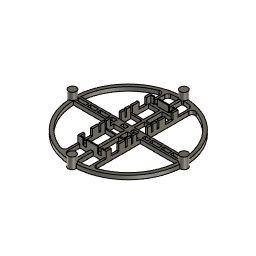
Upper_Bulkhead (Autodesk Fusion 360 design; units mm, degrees)
Autodesk Fusion 360 part; units mm, degrees
sketch "Sketch1" plane through (0, 0, 0) normal (0, 0, 1) x (1, 0, 0)
  circle A0 centre (-0.0658, -87) radius 6
  circle A1 centre (-0.0091, -87) radius 3.15
  circle A2 centre (0.0017, 0.5072) radius 87
  circle A3 centre (-86.9982, 0.5525) radius 3.15
  circle A4 centre (-86.9982, 0.5525) radius 6
  circle A5 centre (87, -0.0091) radius 6
  circle A6 centre (87, -0.0091) radius 3.15
  circle A7 centre (0.0091, 87) radius 3.15
  circle A8 centre (-0.0658, 87) radius 6
  circle A9 centre (0.0017, 0.5072) radius 72.5
  line L0 (-3.9982, 75.5616) -> (4.0018, 75.5616)
  line L1 (4.0018, 75.5616) -> (4.0018, -76.3795)
  line L2 (4.0018, -76.3795) -> (-3.9982, -76.3795)
  line L3 (-3.9982, -76.3795) -> (-3.9982, 75.5616)
  line L4 (-19.9982, 74.1543) -> (-11.9982, 74.1543)
  line L5 (-11.9982, 74.1543) -> (-11.9982, -70.9928)
  line L6 (-11.9982, -70.9928) -> (-19.9982, -70.9928)
  line L7 (-19.9982, -70.9928) -> (-19.9982, 74.1543)
  line L8 (12.0018, -70.9928) -> (20.0018, -70.9928)
  line L9 (20.0018, -70.9928) -> (20.0018, 75.5068)
  line L10 (20.0018, 75.5068) -> (12.0018, 75.5068)
  line L11 (12.0018, 75.5068) -> (12.0018, -70.9928)
  line L12 (0, 2.5) -> (0, 20)
  line L13 (-76.1815, -3) -> (75.8451, -3)
  line L14 (75.8451, -3) -> (75.8451, 0)
  line L15 (75.8451, 0) -> (-76.1815, 0)
  line L16 (-76.1815, 0) -> (-76.1815, -3)
  circle A10 centre (0.0017, 0.5072) radius 82
  line L17 (75.8451, -3) -> (81.9267, -3)
  line L18 (75.8451, 0) -> (82.0002, 0)
  line L19 (20.0018, -70.9928) -> (20.0018, -79.0164)
  line L20 (12.0018, -70.9928) -> (12.0018, -80.61)
  line L21 (-11.9982, -70.9928) -> (-11.9982, -80.61)
  line L22 (-3.9982, -76.3795) -> (-3.9982, -81.3952)
  line L23 (4.0018, -76.3795) -> (4.0018, -81.3952)
  line L24 (-19.9982, -70.9928) -> (-19.9982, -79.0164)
  line L25 (-19.9982, 74.1543) -> (-19.9982, 80.0307)
  line L26 (-11.9982, 74.1543) -> (-11.9982, 81.6244)
  line L27 (-3.9982, 75.5616) -> (-3.9982, 82.4095)
  line L28 (4.0018, 75.5616) -> (4.0018, 82.4095)
  line L29 (12.0018, 75.5068) -> (12.0018, 81.6244)
  line L30 (-76.1815, -3) -> (-81.9232, -3)
  line L31 (-81.9967, 0) -> (-76.1815, 0)
  line L32 (81.8786, 5) -> (-81.8751, 5)
  line L33 (81.6587, 8) -> (-81.6552, 8)
  line L34 (20.0018, 75.5068) -> (20.0018, 80.0307)
  line L35 (66.0018, 0) -> (66.0018, 5)
  line L36 (63.0018, 5) -> (63.0018, 0)
  line L37 (51.0018, 0) -> (51.0018, 5)
  line L38 (48.0018, 0) -> (48.0018, 5)
  line L39 (33.0018, 5) -> (33.0018, 0)
  line L40 (30.0018, 0) -> (30.0018, 5)
  line L41 (-30.0018, 0) -> (-30.0018, 5)
  line L42 (-33.0018, 5) -> (-33.0018, 0)
  line L43 (-48.0018, 0) -> (-48.0018, 5)
  line L44 (-51.0018, 0) -> (-51.0018, 5)
  line L45 (-63.0018, 5) -> (-63.0018, 0)
  line L46 (-66.0018, 0) -> (-66.0018, 5)
  dimension "d15" = 6.3
  dimension "d16" = 12
  dimension "d28" = 6.3
  dimension "d29" = 12
  dimension "d31" = 12
  dimension "d33" = 12
  dimension "d7" = 174
  dimension "d8" = 145
  dimension "d9" = 8
  dimension "d11" = 8
  dimension "d12" = 8
  dimension "d13" = 8
  dimension "d14" = 67
  dimension "d17" = 87
  dimension "d19" = 8
  dimension "d30" = 6.3
  dimension "d32" = 6.3
  dimension "d41" = 3
  dimension "d42" = 3
  dimension "d51" = 164
  dimension "d52" = 5
  dimension "d53" = 3
  dimension "d54" = 3
  dimension "d55" = 3
  dimension "d56" = 3
  dimension "d57" = 15
  dimension "d58" = 15
  dimension "d60" = 10
  constraint concentric A5 A6
  constraint concentric A3 A4
  constraint coincident A3.centre A2
  constraint concentric A2 A9
  constraint horizontal L0
  constraint vertical L1
  constraint horizontal L2
  constraint vertical L3
  constraint horizontal L4
  constraint vertical L5
  constraint horizontal L6
  constraint vertical L7
  constraint coincident A9 L5.end
  constraint horizontal L8
  constraint vertical L9
  constraint horizontal L10
  constraint vertical L11
  constraint coincident A9 L8.start
  constraint horizontal L13
  constraint vertical L14
  constraint horizontal L15
  constraint vertical L16
  constraint concentric A9 A10
  constraint coincident A10 L17.end
  constraint perpendicular L14 L17
  constraint coincident A10 L18.end
  constraint perpendicular L14 L18
  constraint coincident A10 L19.end
  constraint perpendicular L8 L19
  constraint coincident A10 L20.end
  constraint perpendicular L8 L20
  constraint coincident A10 L21.end
  constraint perpendicular L6 L21
  constraint coincident A10 L22.end
  constraint perpendicular L2 L22
  constraint coincident A10 L23.end
  constraint perpendicular L2 L23
  constraint coincident A10 L24.end
  constraint perpendicular L6 L24
  constraint coincident A10 L25.end
  constraint perpendicular L4 L25
  constraint coincident A10 L26.end
  constraint perpendicular L4 L26
  constraint coincident A10 L27.end
  constraint perpendicular L0 L27
  constraint coincident A10 L28.end
  constraint perpendicular L0 L28
  constraint coincident A10 L29.end
  constraint perpendicular L10 L29
  constraint coincident A10 L30.end
  constraint perpendicular L16 L30
  constraint coincident A10 L31.start
  constraint perpendicular L16 L31
  constraint coincident A10 L32.start
  constraint coincident A10 L32.end
  constraint coincident A10 L33.start
  constraint coincident A10 L33.end
  constraint coincident A10 L34.end
  constraint perpendicular L10 L34
  constraint coincident L15 L35.start
  constraint coincident L32 L35.end
  constraint perpendicular L32 L35
  constraint coincident L32 L36.start
  constraint coincident L15 L36.end
  constraint perpendicular L15 L36
  constraint coincident L15 L37.start
  constraint coincident L32 L37.end
  constraint perpendicular L32 L37
  constraint coincident L15 L38.start
  constraint coincident L32 L38.end
  constraint perpendicular L32 L38
  constraint coincident L32 L39.start
  constraint coincident L15 L39.end
  constraint perpendicular L32 L39
  constraint coincident L15 L40.start
  constraint coincident L32 L40.end
  constraint perpendicular L32 L40
  constraint symmetric L12 L35.start L46.start
  constraint symmetric L12 L35.end L46.end
  constraint symmetric L12 L36.start L45.start
  constraint symmetric L12 L36.end L45.end
  constraint symmetric L12 L37.start L44.start
  constraint symmetric L12 L37.end L44.end
  constraint symmetric L12 L38.start L43.start
  constraint symmetric L12 L38.end L43.end
  constraint symmetric L12 L39.start L42.start
  constraint symmetric L12 L39.end L42.end
  constraint symmetric L12 L40.start L41.start
  constraint symmetric L12 L40.end L41.end
  measures "d15" diameter of A6
  measures "d16" diameter of A5
  measures "d28" diameter of A3
  measures "d29" diameter of A4
  measures "d31" diameter of A0
  measures "d33" diameter of A8
  measures "d7" diameter of A2
  measures "d8" diameter of A9
  measures "d9" distance of L1 L3
  measures "d11" distance of L5 L7
  measures "d12" distance of L9 L11
  measures "d13" distance of L3 L5
  measures "d14" distance of A3.centre L7
  measures "d17" distance of origin A3.centre
  measures "d19" distance of L1 L11
  measures "d30" diameter of A1
  measures "d32" diameter of A7
  measures "d41" distance of L13 L15
  measures "d42" distance of origin L13
  measures "d51" diameter of A10
  measures "d52" distance of L15 L32
  measures "d53" distance of L32 L33
  measures "d54" distance of L35 L36
  measures "d55" distance of L37 L38
  measures "d56" distance of L39 L40
  measures "d57" distance of L38 L39
  measures "d58" distance of L35 L37
  measures "d60" distance of L9 L40
extrude "Extrude1" add sketch "Sketch1" along normal blind 6 contours A0 A1 A2 | A0 A1 A2 A10 | A0 A2 A5 A10 | A0 A2 A4 A10 | A0 A10 | A2 A5 A6 A10 | A2 A5 A6 | A2 A3 A4 | A2 A3 A4 A10 | A5 A10 L17 | A2 A4 A8 A10 | A4 A10 L31 | A4 L16 A10 L30 L31 | A5 L14 L17 L18 | A5 A10 L17 L18 | A2 A5 A8 A10 | A2 A7 A8 | A2 A7 A8 A10 | A4 A10 L31 | A5 A10 L18 | A9 L13 L14 L15 | A8 A10 | A9 A10 L32 L33 | A9 L13 L15 L16 | L1 L11 L13 L15 | L9 L11 L13 L15 | L1 L3 L13 L15 | A9 L9 L13 L15 | A9 A10 L32 L33 | L5 L7 L13 L15 | L3 L5 L13 L15 | A9 L7 L32 L33 | A9 L7 L13 L15 | L9 L11 L15 L32 | L1 L3 L15 L32 | A9 L9 L32 L33 | L5 L7 L15 L32 | L15 L32 L45 L46 | L1 L11 L32 L33 | L9 L11 L32 L33 | L1 L12 L32 L33 | L15 L32 L35 L36 | L5 L7 L32 L33 | L3 L5 L32 L33 | L3 L12 L32 L33 | L15 L32 L39 L40 | L15 L32 L41 L42 | L15 L32 L43 L44 | L15 L32 L37 L38
extrude "Extrude2" add sketch "Sketch1" along normal blind 2 contours A0 A1 A2 | A0 A1 A2 A10 | A0 A10 | A2 A5 A6 A10 | A2 A5 A6 | A2 A3 A4 | A2 A3 A4 A10 | A5 A10 L17 | A4 A10 L31 | A5 A10 L17 L18 | A2 A7 A8 | A2 A7 A8 A10 | A4 A10 L31 | A5 A10 L18 | A8 A10
extrude "Extrude3" add sketch "Sketch1" along normal blind 10 contours A0 A1 A2 | A0 A1 A2 A10 | A0 A10 | A2 A5 A6 A10 | A2 A5 A6 | A2 A3 A4 | A2 A3 A4 A10 | A5 A10 L17 | A4 A10 L31 | A5 A10 L17 L18 | A2 A7 A8 | A2 A7 A8 A10 | A4 A10 L31 | A5 A10 L18 | A8 A10
extrude "Extrude4" add sketch "Sketch1" along normal blind 7 from surface at 10 contours A0 A1 A2 | A0 A1 A2 A10 | A0 A10 | A1 A2 | A1 A2 | A2 A5 A6 A10 | A2 A5 A6 | A2 A3 A4 | A2 A3 A4 A10 | A2 A6 | A2 A6 | A5 A10 L17 | A2 A3 | A2 A3 | A4 A10 L31 | A5 A10 L17 L18 | A2 A7 A8 | A2 A7 A8 A10 | A4 A10 L31 | A5 A10 L18 | A2 A7 | A2 A7 | A8 A10
sketch "Sketch2" plane through (0, 0, 6) normal (0, 0, 1) x (-1, 0, 0)
  arc A0 (-81, 0) -> (-81.7986, 3) centre (-87, 0.0091) ccw
  arc A1 (-3.8087, -82.4187) -> (-5.9264, -87.3052) centre (0.0658, -87) ccw
  arc A2 (6.0585, -87.2958) -> (86.7882, -6.5489) centre (-0.0017, -0.5072) ccw
  arc A3 (81.9333, -3.7692) -> (86.7882, -6.5489) centre (86.9982, -0.5525) ccw
  line L0 (-19, 54.5) -> (19, 54.5)
  line L1 (19, 54.5) -> (19, -54.5)
  line L2 (19, -54.5) -> (-19, -54.5)
  line L3 (-19, -54.5) -> (-19, 54.5)
  line L4 (-20.0018, -55.9949) -> (19.9982, -55.9949)
  line L5 (19.9982, -50.9756) -> (19.9982, -55.9949)
  line L6 (19.9982, -50.9756) -> (-20.0018, -50.9756)
  line L7 (-20.0018, -50.9756) -> (-20.0018, -55.9949)
  line L8 (-1.75, 0) -> (-22.5, 0)
  line L9 (19.9982, 50.9756) -> (-20.0018, 50.9756)
  line L10 (-20.0018, 50.9756) -> (-20.0018, 55.9949)
  line L11 (19.9982, 50.9756) -> (19.9982, 55.9949)
  line L12 (-20.0018, 55.9949) -> (19.9982, 55.9949)
  line L13 (-20.0018, -50.9756) -> (-20.0018, 55.9949)
  line L14 (19.9982, 55.9949) -> (19.9982, -50.9756)
  line L15 (19.9982, -55.9949) -> (22.0168, -55.9949)
  line L16 (22.0168, -55.9949) -> (22.0168, 55.9949)
  line L17 (22.0168, 55.9949) -> (19.9982, 55.9949)
  line L18 (0, -1.75) -> (0, -22.5)
  line L19 (-22.0168, -55.9949) -> (-22.0168, 55.9949)
  line L20 (-19.9982, -55.9949) -> (-22.0168, -55.9949)
  line L21 (-22.0168, 55.9949) -> (-19.9982, 55.9949)
  line L22 (-19, -48.1115) -> (-22.0168, -48.1115)
  line L23 (-19, -36.3655) -> (-22.0168, -36.3655)
  line L24 (-19, -32.5412) -> (-22.0168, -32.5412)
  line L25 (-19, -26.0763) -> (-22.0168, -26.0763)
  line L26 (-19, -23.3447) -> (-22.0168, -23.3447)
  line L27 (-19, -16.6067) -> (-22.0168, -16.6067)
  line L28 (-19, -14.6035) -> (-22.0168, -14.6035)
  line L29 (-19, -8.3319) -> (-22.0168, -8.3319)
  line L30 (-19, -6.0084) -> (-22.0168, -6.0084)
  line L31 (19, -32.5412) -> (22.0168, -32.5412)
  line L32 (19, -26.0763) -> (22.0168, -26.0763)
  line L33 (19, -23.3447) -> (22.0168, -23.3447)
  line L34 (19, -36.3655) -> (22.0168, -36.3655)
  line L35 (19, -48.1115) -> (22.0168, -48.1115)
  line L36 (19, -16.6067) -> (22.0168, -16.6067)
  line L37 (19, -14.6035) -> (22.0168, -14.6035)
  line L38 (19, -8.3319) -> (22.0168, -8.3319)
  line L39 (19, -6.0084) -> (22.0168, -6.0084)
  line L40 (-19, 48.1115) -> (-22.0168, 48.1115)
  line L41 (-19, 36.3655) -> (-22.0168, 36.3655)
  line L42 (-19, 32.5412) -> (-22.0168, 32.5412)
  line L43 (-19, 26.0763) -> (-22.0168, 26.0763)
  line L44 (-19, 23.3447) -> (-22.0168, 23.3447)
  line L45 (-19, 16.6067) -> (-22.0168, 16.6067)
  line L46 (-19, 14.6035) -> (-22.0168, 14.6035)
  line L47 (-19, 8.3319) -> (-22.0168, 8.3319)
  line L48 (-19, 6.0084) -> (-22.0168, 6.0084)
  line L49 (19, 6.0084) -> (22.0168, 6.0084)
  line L50 (19, 8.3319) -> (22.0168, 8.3319)
  line L51 (19, 14.6035) -> (22.0168, 14.6035)
  line L52 (19, 16.6067) -> (22.0168, 16.6067)
  line L53 (19, 23.3447) -> (22.0168, 23.3447)
  line L54 (19, 26.0763) -> (22.0168, 26.0763)
  line L55 (19, 32.5412) -> (22.0168, 32.5412)
  line L56 (19, 36.3655) -> (22.0168, 36.3655)
  line L57 (19, 48.1115) -> (22.0168, 48.1115)
  arc A4 (-81.9562, -3.2405) -> (-81.8786, -5) centre (-0.0017, -0.5072) ccw
  line L58 (-81.6587, -8) -> (81.6552, -8)
  line L59 (3.9982, -5) -> (3.9982, 0)
  line L60 (-81, 0) -> (-66.0018, 0)
  line L61 (11.9982, 0) -> (11.9982, -5)
  line L62 (11.9982, -5) -> (3.9982, -5)
  line L63 (-51.0018, -5) -> (-63.0018, -5)
  line L64 (19.9982, -5) -> (19.9982, 0)
  line L65 (81.9232, 3) -> (-81.7986, 3)
  line L66 (-30.0018, 0) -> (-20.0018, 0)
  line L67 (-20.0018, 0) -> (-20.0018, -5)
  line L68 (-12.0018, -5) -> (-12.0018, 0)
  line L69 (-12.0018, 0) -> (-4.0018, 0)
  line L70 (-4.0018, 0) -> (-4.0018, -5)
  line L71 (-4.0018, -5) -> (-12.0018, -5)
  line L72 (19.9982, 0) -> (30.0018, 0)
  line L73 (81.8751, -5) -> (66.0018, -5)
  arc A5 (2.3665, 81.4586) -> (6.0229, 86.284) centre (0.0658, 87) ccw
  arc A6 (-86.8289, -5.9884) -> (-5.9264, -87.3052) centre (-0.0017, -0.5072) ccw
  arc A7 (86.7945, 5.444) -> (6.0229, 86.284) centre (-0.0017, -0.5072) ccw
  line L74 (-63.0018, -5) -> (-63.0018, 0)
  line L75 (-51.0018, 0) -> (-51.0018, -5)
  line L76 (-48.0018, -5) -> (-48.0018, 0)
  line L77 (-48.0018, 0) -> (-33.0018, 0)
  line L78 (-33.0018, 0) -> (-33.0018, -5)
  line L79 (-66.0018, 0) -> (-66.0018, -5)
  line L80 (-30.0018, -5) -> (-30.0018, 0)
  arc A8 (81.9232, 3) -> (2.3665, 81.4586) centre (-0.0017, -0.5072) ccw
  line L81 (51.0018, -5) -> (51.0018, 0)
  line L82 (51.0018, 0) -> (63.0018, 0)
  line L83 (63.0018, 0) -> (63.0018, -5)
  line L84 (63.0018, -5) -> (51.0018, -5)
  line L85 (66.0018, 0) -> (81.0237, 0)
  line L86 (66.0018, -5) -> (66.0018, 0)
  line L87 (48.0018, -5) -> (33.0018, -5)
  line L88 (33.0018, -5) -> (33.0018, 0)
  line L89 (33.0018, 0) -> (48.0018, 0)
  line L90 (48.0018, 0) -> (48.0018, -5)
  line L91 (30.0018, 0) -> (30.0018, -5)
  line L92 (30.0018, -5) -> (19.9982, -5)
  arc A9 (3.9332, -82.4127) -> (81.6552, -8) centre (-0.0017, -0.5072) ccw
  line L93 (-63.0018, 0) -> (-51.0018, 0)
  line L94 (-33.0018, -5) -> (-48.0018, -5)
  line L95 (-66.0018, -5) -> (-81.8786, -5)
  line L96 (-20.0018, -5) -> (-30.0018, -5)
  arc A10 (-86.8289, -5.9884) -> (-81.9562, -3.2405) centre (-87, 0.0091) ccw
  arc A11 (-81.6587, -8) -> (-3.8087, -82.4187) centre (-0.0017, -0.5072) ccw
  arc A12 (6.0585, -87.2958) -> (3.9332, -82.4127) centre (0.0658, -87) ccw
  arc A13 (81.8751, -5) -> (81.9333, -3.7692) centre (-0.0017, -0.5072) ccw
  arc A14 (86.7945, 5.444) -> (81.0237, 0) centre (86.9982, -0.5525) ccw
  line L97 (3.9982, 0) -> (11.9982, 0)
  line L98 (-19, -54.5) -> (-19, -80.276)
  line L99 (-22.0168, -55.9949) -> (-22.0168, -79.4966)
  line L100 (22.0168, -55.9949) -> (22.0168, -79.4957)
  line L101 (19, -54.5) -> (19, -80.2752)
  line L102 (22.0168, 55.9949) -> (22.0168, 78.4813)
  line L103 (19, 54.5) -> (19, 79.2608)
  line L104 (-19, 54.5) -> (-19, 79.2608)
  line L105 (-22.0168, 55.9949) -> (-22.0168, 79.2608)
  line L106 (-22.0168, 79.2608) -> (-19, 79.2608)
  line L107 (-2, 6.1969) -> (-2, -11.5663)
  line L108 (2, 6.1969) -> (2, -11.6219)
  line L109 (2, -11.6219) -> (-2, -11.5663)
  line L110 (-2, 6.1969) -> (2, 6.1969)
  line L111 (-2, -11.5663) -> (1.9507, -11.5663)
  line L112 (1.9507, -11.5663) -> (1.9507, -82.4127)
  line L113 (1.9507, -82.4127) -> (-2, -82.4127)
  line L114 (-2, -82.4127) -> (-2, -11.5663)
  line L115 (-2, 6.1969) -> (2.3665, 6.1969)
  line L116 (2.3665, 6.1969) -> (2.3665, 81.4586)
  line L117 (2.3665, 81.4586) -> (-2, 81.4586)
  line L118 (-2, 81.4586) -> (-2, 6.1969)
  line L119 (-19, -26.0763) -> (19, -26.0763)
  line L120 (19, -23.3447) -> (-19, -23.3447)
  line L121 (-19, 14.6035) -> (19, 14.6035)
  line L122 (19, 16.6067) -> (-19, 16.6067)
  line L123 (14.149, -54.5) -> (14.149, -55.9949)
  line L124 (8.7018, -55.9949) -> (8.7018, -54.5)
  line L125 (-14.149, -54.5) -> (-14.149, -55.9949)
  line L126 (-8.7018, -55.9949) -> (-8.7018, -54.5)
  dimension "d43" = 38
  dimension "d44" = 19
  dimension "d45" = 54.5
  dimension "d46" = 54.5
  dimension "d61" = 2
  dimension "d62" = 4
  constraint horizontal L0
  constraint vertical L1
  constraint horizontal L2
  constraint vertical L3
  constraint perpendicular L4 L5
  constraint symmetric L4.start L8 L10.end
  constraint symmetric L4.end L8 L11.end
  constraint symmetric L5.start L8 L9.start
  constraint symmetric L6.end L8 L9.end
  constraint perpendicular L12 L13
  constraint perpendicular L15 L16
  constraint perpendicular L16 L17
  constraint symmetric L4.end L18 L20.start
  constraint symmetric L11.end L18 L21.end
  constraint symmetric L15.end L18 L19.start
  constraint symmetric L16.end L18 L19.end
  constraint coincident L3 L22.start
  constraint coincident L19 L22.end
  constraint perpendicular L19 L22
  constraint coincident L3 L23.start
  constraint coincident L19 L23.end
  constraint perpendicular L19 L23
  constraint coincident L3 L24.start
  constraint coincident L19 L24.end
  constraint perpendicular L19 L24
  constraint coincident L3 L25.start
  constraint coincident L19 L25.end
  constraint perpendicular L19 L25
  constraint coincident L3 L26.start
  constraint coincident L19 L26.end
  constraint perpendicular L19 L26
  constraint coincident L3 L27.start
  constraint coincident L19 L27.end
  constraint perpendicular L19 L27
  constraint coincident L3 L28.start
  constraint coincident L19 L28.end
  constraint perpendicular L19 L28
  constraint coincident L3 L29.start
  constraint coincident L19 L29.end
  constraint perpendicular L19 L29
  constraint coincident L3 L30.start
  constraint coincident L19 L30.end
  constraint perpendicular L19 L30
  constraint symmetric L18 L22.start L35.start
  constraint symmetric L18 L22.end L35.end
  constraint symmetric L18 L23.start L34.start
  constraint symmetric L18 L23.end L34.end
  constraint symmetric L18 L24.start L31.start
  constraint symmetric L18 L24.end L31.end
  constraint symmetric L18 L25.start L32.start
  constraint symmetric L18 L25.end L32.end
  constraint symmetric L18 L26.start L33.start
  constraint symmetric L18 L26.end L33.end
  constraint symmetric L18 L27.start L36.start
  constraint symmetric L18 L27.end L36.end
  constraint symmetric L18 L28.start L37.start
  constraint symmetric L18 L28.end L37.end
  constraint symmetric L18 L29.start L38.start
  constraint symmetric L18 L29.end L38.end
  constraint symmetric L18 L30.start L39.start
  constraint symmetric L18 L30.end L39.end
  constraint symmetric L8 L22.start L40.start
  constraint symmetric L8 L22.end L40.end
  constraint symmetric L8 L23.start L41.start
  constraint symmetric L8 L23.end L41.end
  constraint symmetric L8 L24.start L42.start
  constraint symmetric L8 L24.end L42.end
  constraint symmetric L8 L25.start L43.start
  constraint symmetric L8 L25.end L43.end
  constraint symmetric L8 L26.start L44.start
  constraint symmetric L8 L26.end L44.end
  constraint symmetric L8 L27.start L45.start
  constraint symmetric L8 L27.end L45.end
  constraint symmetric L8 L28.start L46.start
  constraint symmetric L8 L28.end L46.end
  constraint symmetric L8 L29.start L47.start
  constraint symmetric L8 L29.end L47.end
  constraint symmetric L8 L30.start L48.start
  constraint symmetric L8 L30.end L48.end
  constraint symmetric L8 L31.start L55.start
  constraint symmetric L8 L31.end L55.end
  constraint symmetric L8 L32.start L54.start
  constraint symmetric L8 L32.end L54.end
  constraint symmetric L8 L33.start L53.start
  constraint symmetric L8 L33.end L53.end
  constraint symmetric L8 L34.start L56.start
  constraint symmetric L8 L34.end L56.end
  constraint symmetric L8 L35.start L57.start
  constraint symmetric L8 L35.end L57.end
  constraint symmetric L8 L36.start L52.start
  constraint symmetric L8 L36.end L52.end
  constraint symmetric L8 L37.start L51.start
  constraint symmetric L8 L37.end L51.end
  constraint symmetric L8 L38.start L50.start
  constraint symmetric L8 L38.end L50.end
  constraint symmetric L8 L39.start L49.start
  constraint symmetric L8 L39.end L49.end
  constraint coincident A11 L98.end
  constraint perpendicular L2 L98
  constraint coincident A11 L99.end
  constraint perpendicular L20 L99
  constraint coincident A9 L100.end
  constraint perpendicular L15 L100
  constraint coincident A9 L101.end
  constraint perpendicular L4 L101
  constraint coincident A8 L102.end
  constraint perpendicular L17 L102
  constraint coincident A8 L103.end
  constraint perpendicular L12 L103
  constraint perpendicular L12 L104
  constraint perpendicular L21 L105
  constraint perpendicular L104 L106
  constraint perpendicular L58 L107
  constraint perpendicular L58 L108
  constraint perpendicular L108 L110
  constraint horizontal L111
  constraint vertical L112
  constraint horizontal L113
  constraint vertical L114
  constraint horizontal L115
  constraint vertical L116
  constraint horizontal L117
  constraint vertical L118
  constraint coincident A5.start A8.end
  constraint coincident L2 L123.start
  constraint coincident L4 L123.end
  constraint perpendicular L4 L123
  constraint coincident L4 L124.start
  constraint coincident L2 L124.end
  constraint perpendicular L2 L124
  constraint symmetric L18 L123.start L125.start
  constraint symmetric L18 L123.end L125.end
  constraint symmetric L18 L124.start L126.start
  constraint symmetric L18 L124.end L126.end
  measures "d43" distance of L0.start L0.end
  measures "d44" distance of origin L1
  measures "d45" distance of origin L0
  measures "d46" distance of origin L2
  measures "d61" distance of origin L108
  measures "d62" distance of L107 L108
extrude "Extrude7" add sketch "Sketch2" 1 faces at (-19.8025, -80.6074, 6) against normal blind 6 contours L8 L13 L19 L65 L66 | L13 L19 L48 L65 | L8 L13 L19 L66 L67 L96 | L13 L19 L47 L48 | L3 L8 L13 L65 | L3 L13 L48 L65 | L3 L8 L13 L30 L67 | L13 L19 L30 L96 | L13 L19 L46 L47 | L3 L13 L47 L48 | L13 L19 L30 L58 | L13 L19 L45 L46 | L3 L13 L46 L47 | L65 L107 L108 L110 L115 | L58 L65 L107 L108 | L3 L13 L30 L58 | L13 L19 L29 L58 | L13 L19 L44 L45 | L3 L13 L45 L46 | L110 L115 L116 L118 L121 | L3 L13 L29 L58 | L13 L19 L28 L29 | L13 L19 L43 L44 | L3 L13 L44 L45 | L3 L118 L121 L122 | L1 L14 L39 L64 L65 | L1 L14 L49 L65 | L18 L58 L108 L109 L111 L112 | L116 L118 L121 L122 | L18 L58 L107 L111 | L3 L13 L28 L29 | L13 L19 L27 L28 | L4 L20 A11 L98 L99 | L13 L19 L42 L43 | L3 L13 L43 L44 | L1 L14 L49 L50 | L1 L14 L39 L58 | L14 L16 L65 L72 | L14 L16 L49 L65 | L1 L14 L38 L58 | L9 L116 L118 L122 | L1 L116 L121 L122 | L18 L109 L111 | L109 L112 L114 L120 | L3 L13 L27 L28 | L13 L19 L26 L27 | L7 L13 L19 L20 L22 | L13 L19 L41 L42 | L3 L13 L42 L43 | L1 L14 L50 L51 | L14 L16 L49 L50 | L14 L16 L39 L58 | L14 L16 L39 L92 | L14 L16 L64 L72 L92 | A2 A3 L16 L58 L65 L72 L73 A5 A7 A8 L85 L86 L91 L92 A9 A12 A13 A14 | L18 L109 L111 L112 | L1 L14 L37 L38 | L14 L16 L38 L58 | L0 L9 L116 L118 | L0 L3 L9 L118 | L1 L14 L51 L52 | L112 L114 L119 L120 | L3 L114 L119 L120 | L2 L4 L98 L125 | L3 L4 L6 L7 L20 L98 | L3 L13 L26 L27 | L13 L19 L25 L26 | L13 L19 L22 L23 | L13 L19 L40 L41 | L3 L13 L41 L42 | L14 L16 L50 L51 | L1 L14 L36 L37 | L14 L16 L37 L38 | L1 L112 L119 L120 | L0 L1 L9 L116 | L3 L9 L10 L12 L13 L21 L104 | L3 L9 L13 L40 | L0 L12 L116 L118 | L0 L12 L104 L118 | L1 L14 L52 L53 | L14 L16 L51 L52 | L6 L112 L114 L119 | L3 L13 L25 L26 | L2 L4 L125 L126 | L2 L3 L6 L114 | L13 L19 L24 L25 | L13 L19 L23 L24 | L3 L6 L13 L22 | L3 L13 L22 L23 | L10 L13 L19 L21 L40 | L3 L13 L40 L41 | L12 L17 A8 L102 L103 | L1 L14 L33 L36 | L14 L16 L36 L37 | L1 L14 L32 L33 | L1 L9 L14 L57 | L1 L9 L11 L12 L14 L103 | L0 L12 L103 L116 | L12 L116 L117 L118 | L1 L14 L53 L54 | L14 L16 L52 L53 | L2 L6 L112 L114 | L3 L13 L24 L25 | L2 L4 L114 L126 | L3 L13 L23 L24 | L12 L21 L104 L105 L106 | L11 L14 L16 L17 L57 | L14 L16 L33 L36 | L4 L15 A9 L100 L101 | L1 L2 L6 L112 | L1 L14 L31 L32 | L14 L16 L32 L33 | L1 L14 L56 L57 | L1 L14 L54 L55 | L14 L16 L53 L54 | L2 L4 L112 L114 | L4 L112 L113 L114 | L14 L16 L56 L57 | L5 L14 L15 L16 L35 | L1 L4 L5 L6 L101 | L1 L6 L14 L35 | L2 L4 L112 L124 | L1 L14 L31 L34 | L14 L16 L31 L32 | L1 L14 L55 L56 | L14 L16 L54 L55 | L14 L16 L55 L56 | L2 L4 L101 L123 | L14 L16 L34 L35 | L1 L14 L34 L35 | L2 L4 L123 L124 | L14 L16 L31 L34
extrude "Extrude8" add sketch "Sketch2" along normal blind 10 contours L13 L19 L28 L29 | L3 L13 L28 L29 | L13 L19 L26 L27 | L7 L13 L19 L20 L22 | L1 L14 L37 L38 | L2 L4 L98 L125 | L3 L4 L6 L7 L20 L98 | L3 L13 L26 L27 | L14 L16 L37 L38 | L13 L19 L24 L25 | L13 L19 L23 L24 | L3 L6 L13 L22 | L1 L14 L33 L36 | L3 L13 L24 L25 | L2 L4 L114 L126 | L3 L13 L23 L24 | L14 L16 L33 L36 | L1 L14 L31 L32 | L2 L4 L112 L114 | L5 L14 L15 L16 L35 | L1 L4 L5 L6 L101 | L1 L6 L14 L35 | L2 L4 L112 L124 | L1 L14 L31 L34 | L14 L16 L31 L32 | L2 L4 L101 L123 | L14 L16 L31 L34
mirror "Mirror1" about plane through (0, 0, 0) normal (0, 1, 0) of "Extrude8"
fillet "Fillet1" radius 5 10 edges at (19, 80.276, 3) (22.0168, 79.4966, 3) (-19, 80.2752, 3) (-22.0168, 79.4957, 3) (-2.3665, -81.4586, 3) (19, -79.2608, 3) (-22.0168, -78.4813, 3) (-19, -79.2608, 3) (2, -81.3668, 3) (22.0168, -78.4823, 3)
